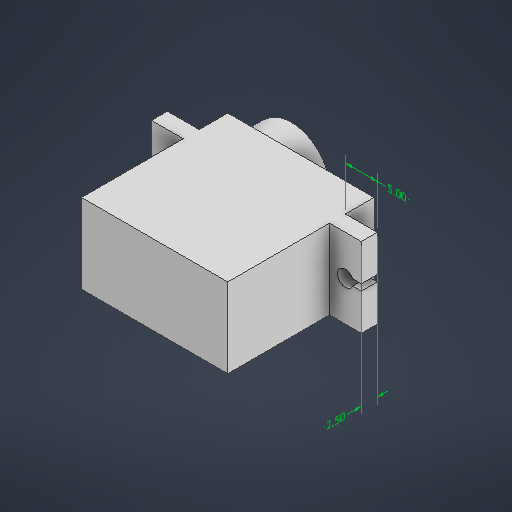
# Autodesk Inventor part: Micro servo
Saved by Autodesk Inventor 2026.2 (Build 302298000, 298)
## iProperties
Created: 2026-01-19
Part Number: Micro servo
Material: Generic
Document SubType Name: Modeling
Designer: ASUS
Density: 1 g/cm^3
Appearance: Default
Author: ASUS
Autodesk Inventor part; units mm, degrees
ref_plane "YZ Plane" through (0, 0, 0) normal (1, 0, 0) x (0, 1, 0)
ref_plane "XZ Plane" through (0, 0, 0) normal (0, 1, 0) x (-1, 0, 0)
ref_plane "XY Plane" through (0, 0, 0) normal (0, 0, 1) x (1, 0, 0)
sketch "Sketch1" plane through (0, 0, 0) normal (0, 1, 0) x (-1, 0, 0)
  line L0 (0, 0) -> (-23, 0)
  line L1 (-23, 0) -> (-23, 23)
  line L2 (-23, 23) -> (0, 23)
  line L3 (0, 23) -> (0, 0)
  line L4 (-23, 0) -> (-23, 7)
  line L5 (-23, 7) -> (-28, 7)
  line L6 (-28, 7) -> (-28, 4.5)
  line L7 (-28, 4.5) -> (-23, 4.5)
  line L8 (0, 7) -> (5, 7)
  line L9 (5, 7) -> (5, 4.5)
  line L10 (5, 4.5) -> (0, 4.5)
  dimension "d0" = 23
  dimension "d1" = 23
  dimension "d2" = 7
  dimension "d3" = 5
  dimension "d4" = 2.5
  constraints: 22 end point, 4 perpendicular, 2 parallel, 2 point on line, 1 horizontal
  measures "d0" distance of L1.end L2.end
  measures "d1" distance of L0.end L1.end
  measures "d2" distance of L0.end L4.end
  measures "d3" distance of L4.end L5.end
  measures "d4" distance of L5.end L6.end
extrude "Extrusion1" add sketch "Sketch1" along normal blind 12.5
sketch "Sketch2" plane through (23, 0, 0) normal (0, 0, -1) x (-1, 0, 0)
  line L0 (23, 0) -> (23, 6.25)
  arc A0 (11.2156, 4.6561) -> (11.2214, 7.865) centre (17, 6.25) ccw
  arc A1 (11.2214, 7.865) -> (11.2156, 4.6561) centre (10.0244, 6.2627) ccw
  constraints: 5 point on circle, 2 centre point, 2 end point
extrude "Extrusion2" add sketch "Sketch2" along normal blind 4
sketch "Sketch3" plane through (28, 0, 4.5) normal (0, 0, -1) x (-1, 0, 0)
  line L0 (0, 0) -> (0, 12.5) projected
  line L1 (0, 6.25) -> (2.5, 6.25)
  circle A0 centre (2.5, 6.25) radius 1.25
  point P0 (28, 0)
  dimension "d11" = 2.5
  dimension "d12" = 2.5
  constraints: 2 end point, 1 centre point, 1 coincident, 1 horizontal, 1 midpoint
  measures "d11" distance of L1.start L1.end
  measures "d12" diameter of A0
extrude "Extrusion3" cut sketch "Sketch3" against normal blind 2.5
sketch "Sketch4" plane through (28, 0, 4.5) normal (0, 0, -1) x (-1, 0, 0)
  circle A0 centre (2.5, 6.25) radius 1.25 projected
  line L0 (0, 0) -> (0, 12.5) projected
  line L1 (1.25, 5.75) -> (0, 5.75)
  line L2 (1.25, 6.75) -> (0, 6.75)
  line L3 (1.25, 6.75) -> (1.3544, 6.75)
  line L4 (1.25, 5.75) -> (1.3544, 5.75)
  line L5 (0, 6.75) -> (0, 5.75)
  arc A1 (1.25, 6.25) -> (1.3544, 6.75) centre (2.5, 6.25) ccw
  point P0 (28, 0)
  constraints: 10 end point, 6 point on circle, 2 perpendicular, 1 centre point, 1 horizontal, 1 point on line
extrude "Extrusion4" cut sketch "Sketch4" against normal blind 2.5 contours A0 L4 L1 L0 L2 L3
sketch "Sketch5" plane through (28, 0, 4.5) normal (0, 0, -1) x (-1, 0, 0)
  line L0 (5, 0) -> (28, 0) projected
  line L1 (16.5, 0) -> (16.5, 12.5)
  line L2 (5, 12.5) -> (28, 12.5) projected
  arc A0 (1.3544, 5.75) -> (1.3544, 6.75) centre (2.5, 6.25) ccw projected
  line L3 (1.3544, 6.75) -> (0, 6.75) projected
  line L4 (1.3544, 6.75) -> (0, 6.75)
  line L5 (0, 6.75) -> (0, 5.75)
  line L6 (0, 5.75) -> (1.3544, 5.75)
  arc A1 (31.6456, 6.75) -> (31.6456, 5.75) centre (30.5, 6.25) ccw
  line L7 (31.6456, 6.75) -> (33, 6.75)
  line L8 (33, 6.75) -> (33, 5.75)
  line L9 (33, 5.75) -> (31.6456, 5.75)
  constraints: 14 end point, 5 symmetric about line, 2 midpoint, 2 perpendicular, 2 point on circle, 1 centre point, 1 horizontal, 1 other
extrude "Extrusion5" cut sketch "Sketch5" against normal blind 2.5 contours L7 L8 L9 A1
body "Solid1"
